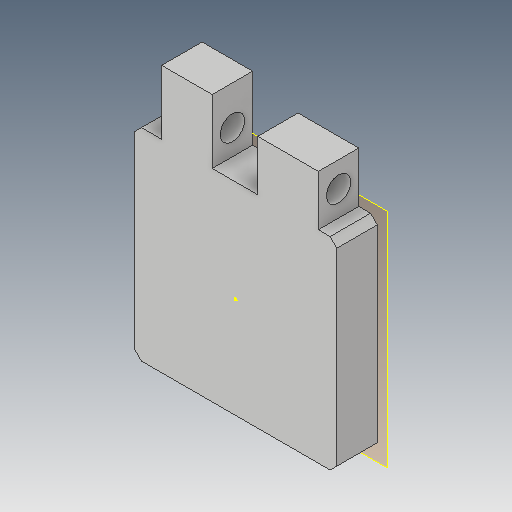
# Autodesk Inventor part: 00_XY_stage-CHUO_SEIKI_LD-647-R1-Middle
Saved by Autodesk Inventor 2019 (Build 230136000, 136)
## iProperties
Created: 2019-05-02
Part Number: 00_XY_stage-CHUO_SEIKI_LD-647-R1-Middle
Material: Generic
Document SubType Name: Modeling
Designer: diederichbenedict
Density: 1 g/cm^3
Appearance: Default
Author: diederichbenedict
Autodesk Inventor part; units mm, degrees
ref_plane "YZ Plane" through (0, 0, 0) normal (1, 0, 0) x (0, 1, 0)
ref_plane "XZ Plane" through (0, 0, 0) normal (0, 1, 0) x (-1, 0, 0)
ref_plane "XY Plane" through (0, 0, 0) normal (0, 0, 1) x (1, 0, 0)
ref_plane "Work Plane1" through (0, 0, 0) normal (0, 0, 1) x (1, 0, 0)
sketch "Sketch1" plane through (0, 0, 0) normal (0, 0, 1) x (1, 0, 0)
  circle A0 centre (17.5, 17.5) radius 1.95 projected
  circle A1 centre (17.5, -17.5) radius 1.95 projected
  circle A2 centre (-17.5, -17.5) radius 1.95 projected
  circle A3 centre (-17.5, 17.5) radius 1.95 projected
  circle A4 centre (0, 0) radius 7.5 projected
  line L0 (-30, 28) -> (-28, 30) projected
  line L1 (-30, -28) -> (-30, 28) projected
  line L2 (-28, -30) -> (-30, -28) projected
  line L3 (28, -30) -> (-28, -30) projected
  line L4 (30, -28) -> (28, -30) projected
  line L5 (30, 28) -> (30, -28) projected
  line L6 (28, 30) -> (30, 28) projected
  line L7 (-28, 30) -> (28, 30) projected
extrude "Extrusion1" add sketch "Sketch1" along normal blind 12 contours A0 | A1 | A2 | A3 | A4 | L0 L7 L6 L5 L4 L3 L2 L1
sketch "Sketch2" plane through (0, 0, 12) normal (0, 0, 1) x (1, 0, 0)
  point P0 (0, 0)
sketch "Sketch5" plane through (0, 0, 0) normal (0, 0, -1) x (-1, 0, 0)
  line L0 (49, -22) -> (49, -7)
  line L1 (30, -28) -> (30, 28) projected
  line L2 (45, 6.5) -> (45, 24.5)
  line L3 (49, -7) -> (30, -7)
  line L4 (30, -7) -> (30, -22)
  line L5 (30, -22) -> (49, -22)
  line L6 (49, -22) -> (49, -7)
  line L7 (45, 6.5) -> (30, 6.5)
  line L8 (30, 6.5) -> (30, 24.5)
  line L9 (30, 24.5) -> (45, 24.5)
  line L10 (45, 24.5) -> (45, 6.5)
  line L11 (22, 49) -> (7, 49)
  line L12 (-6.5, 45) -> (-24.5, 45)
  line L13 (7, 49) -> (7, 30)
  line L14 (7, 30) -> (22, 30)
  line L15 (22, 30) -> (22, 49)
  line L16 (22, 49) -> (7, 49)
  line L17 (-6.5, 45) -> (-6.5, 30)
  line L18 (-6.5, 30) -> (-24.5, 30)
  line L19 (-24.5, 30) -> (-24.5, 45)
  line L20 (-24.5, 45) -> (-6.5, 45)
  point P0 (0, 0)
  point P1 (-28, 30)
  dimension "d12" = 90
  constraints: 40 end point, 4 parallel, 2 horizontal, 2 perpendicular, 2 point on line, 2 vertical, 26 other
extrude "Extrusion4" add sketch "Sketch5" against normal up to surface (12 mm away) contours L15 L14 L13 L11 | L17 L18 L19 L12
sketch "Sketch6" plane through (24.5, 30, 0) normal (1, 0, 0) x (0, 0, -1)
  line L0 (-12, 0) -> (-12, 15) projected
  line L1 (0, 0) -> (-12, 0) projected
  line L2 (0, 0) -> (0, 15) projected
  line L3 (0, 15) -> (-12, 15) projected
  circle A0 centre (-6, 7.5) radius 3.6127
  point P0 (0, -30)
  constraints: 1 centre point
extrude "Extrusion5" cut sketch "Sketch6" against normal through all contours A0
body "Solid1"
